Autodesk Inventor part; units mm, degrees
(part 2 of 2)
  line L89 (15.0406, 0.6529) -> (15.0498, 0.6529)
  line L90 (15.0498, 0.6529) -> (15.0498, 0.478)
  spline S139 degree 2 poles (15.0498, 0.478) (15.022, 0.4666) (14.9377, 0.4337) (14.9047, 0.4244) knots 0 0 0 1 2 2 2
  spline S140 degree 2 poles (14.9047, 0.4244) (14.8584, 0.4111) (14.7822, 0.3977) (14.7246, 0.3977) knots 0 0 0 1 2 2 2
  spline S141 degree 2 poles (14.9109, 1.0018) (14.9088, 1.0666) (14.8821, 1.1613) (14.8563, 1.1932) knots 0 0 0 1 2 2 2
  spline S142 degree 2 poles (14.8563, 1.1932) (14.8286, 1.2293) (14.7411, 1.2673) (14.6762, 1.2673) knots 0 0 0 1 2 2 2
  spline S143 degree 2 poles (14.6762, 1.2673) (14.6124, 1.2673) (14.5229, 1.2293) (14.4858, 1.1922) knots 0 0 0 1 2 2 2
  spline S144 degree 2 poles (14.4858, 1.1922) (14.4498, 1.1541) (14.4128, 1.0625) (14.4076, 1.0018) knots 0 0 0 1 2 2 2
  line L91 (14.4076, 1.0018) -> (14.9109, 1.0018)
  line L92 (16.7099, 0.4193) -> (16.5411, 0.4193)
  line L93 (16.5411, 0.4193) -> (16.5411, 1.0409)
  line L94 (16.5411, 1.0409) -> (15.9565, 1.0409)
  line L95 (15.9565, 1.0409) -> (15.9565, 0.4193)
  line L96 (15.9565, 0.4193) -> (15.7878, 0.4193)
  line L97 (15.7878, 0.4193) -> (15.7878, 1.6893)
  line L98 (15.7878, 1.6893) -> (15.9565, 1.6893)
  line L99 (15.9565, 1.6893) -> (15.9565, 1.1912)
  line L100 (15.9565, 1.1912) -> (16.5411, 1.1912)
  line L101 (16.5411, 1.1912) -> (16.5411, 1.6893)
  line L102 (16.5411, 1.6893) -> (16.7099, 1.6893)
  line L103 (16.7099, 1.6893) -> (16.7099, 0.4193)
  line L104 (17.1185, 0.4193) -> (16.9579, 0.4193)
  line L105 (16.9579, 0.4193) -> (16.9579, 1.3723)
  line L106 (16.9579, 1.3723) -> (17.1185, 1.3723)
  line L107 (17.1185, 1.3723) -> (17.1185, 0.4193)
  line L108 (17.1298, 1.5308) -> (16.9476, 1.5308)
  line L109 (16.9476, 1.5308) -> (16.9476, 1.6975)
  line L110 (16.9476, 1.6975) -> (17.1298, 1.6975)
  line L111 (17.1298, 1.6975) -> (17.1298, 1.5308)
  spline S145 degree 2 poles (17.3881, 0.267) (17.4046, 0.2598) (17.4674, 0.2371) (17.5075, 0.2279) knots 0 0 0 1 2 2 2
  spline S146 degree 2 poles (17.5075, 0.2279) (17.5518, 0.2166) (17.6269, 0.2032) (17.6711, 0.2032) knots 0 0 0 1 2 2 2
  spline S147 degree 2 poles (17.6711, 0.2032) (17.7452, 0.2032) (17.8482, 0.2423) (17.877, 0.2773) knots 0 0 0 1 2 2 2
  spline S148 degree 2 poles (17.877, 0.2773) (17.9048, 0.3123) (17.9264, 0.4039) (17.9264, 0.4625) knots 0 0 0 1 2 2 2
  line L112 (17.9264, 0.4625) -> (17.9264, 0.5459)
  spline S149 degree 2 poles (17.9264, 0.5459) (17.8615, 0.4893) (17.737, 0.4358) (17.6434, 0.4358) knots 0 0 0 1 2 2 2
  spline S150 degree 2 poles (17.6434, 0.4358) (17.4807, 0.4358) (17.2883, 0.6776) (17.2883, 0.9051) knots 0 0 0 1 2 2 2
  spline S151 degree 2 poles (17.2883, 0.9051) (17.2883, 1.0234) (17.3552, 1.2066) (17.4108, 1.2715) knots 0 0 0 1 2 2 2
  spline S152 degree 2 poles (17.4108, 1.2715) (17.4643, 1.3322) (17.6114, 1.3991) (17.6897, 1.3991) knots 0 0 0 1 2 2 2
  spline S153 degree 2 poles (17.6897, 1.3991) (17.7638, 1.3991) (17.8718, 1.3641) (17.9264, 1.3322) knots 0 0 0 1 2 2 2
  line L113 (17.9264, 1.3322) -> (17.9356, 1.3723)
  line L114 (17.9356, 1.3723) -> (18.0869, 1.3723)
  line L115 (18.0869, 1.3723) -> (18.0869, 0.5284)
  spline S154 degree 2 poles (18.0869, 0.5284) (18.0869, 0.2855) (17.8759, 0.0591) (17.6588, 0.0591) knots 0 0 0 1 2 2 2
  spline S155 degree 2 poles (17.6588, 0.0591) (17.5888, 0.0591) (17.4427, 0.0817) (17.3799, 0.1003) knots 0 0 0 1 2 2 2
  line L116 (17.3799, 0.1003) -> (17.3799, 0.267)
  line L117 (17.3799, 0.267) -> (17.3881, 0.267)
  line L118 (17.9264, 0.6776) -> (17.9264, 1.2015)
  spline S156 degree 2 poles (17.9264, 1.2015) (17.8667, 1.2303) (17.7658, 1.255) (17.7154, 1.255) knots 0 0 0 1 2 2 2
  spline S157 degree 2 poles (17.7154, 1.255) (17.5939, 1.255) (17.454, 1.0759) (17.454, 0.9082) knots 0 0 0 1 2 2 2
  spline S158 degree 2 poles (17.454, 0.9082) (17.454, 0.7497) (17.56, 0.584) (17.6794, 0.584) knots 0 0 0 1 2 2 2
  spline S159 degree 2 poles (17.6794, 0.584) (17.7422, 0.584) (17.8739, 0.6334) (17.9264, 0.6776) knots 0 0 0 1 2 2 2
  line L119 (19.0677, 0.4193) -> (18.9072, 0.4193)
  line L120 (18.9072, 0.4193) -> (18.9072, 0.9627)
  spline S160 degree 2 poles (18.9072, 0.9627) (18.9072, 1.0286) (18.8948, 1.1418) (18.8763, 1.1757) knots 0 0 0 1 2 2 2
  spline S161 degree 2 poles (18.8763, 1.1757) (18.8567, 1.2118) (18.7868, 1.2468) (18.7271, 1.2468) knots 0 0 0 1 2 2 2
  spline S162 degree 2 poles (18.7271, 1.2468) (18.6674, 1.2468) (18.5408, 1.1829) (18.4801, 1.1315) knots 0 0 0 1 2 2 2
  line L121 (18.4801, 1.1315) -> (18.4801, 0.4193)
  line L122 (18.4801, 0.4193) -> (18.3195, 0.4193)
  line L123 (18.3195, 0.4193) -> (18.3195, 1.7459)
  line L124 (18.3195, 1.7459) -> (18.4801, 1.7459)
  line L125 (18.4801, 1.7459) -> (18.4801, 1.2663)
  spline S163 degree 2 poles (18.4801, 1.2663) (18.5521, 1.3311) (18.691, 1.3991) (18.7693, 1.3991) knots 0 0 0 1 2 2 2
  spline S164 degree 2 poles (18.7693, 1.3991) (18.9092, 1.3991) (19.0677, 1.2138) (19.0677, 1.0378) knots 0 0 0 1 2 2 2
  line L126 (19.0677, 1.0378) -> (19.0677, 0.4193)
  spline S165 degree 2 poles (20.205, 0.3967) (20.0671, 0.3967) (19.8736, 0.4543) (19.7881, 0.4955) knots 0 0 0 1 2 2 2
  line L127 (19.7881, 0.4955) -> (19.7881, 0.7075)
  line L128 (19.7881, 0.7075) -> (19.8005, 0.7075)
  spline S166 degree 2 poles (19.8005, 0.7075) (19.8839, 0.6292) (20.0948, 0.5428) (20.1926, 0.5428) knots 0 0 0 1 2 2 2
  spline S167 degree 2 poles (20.1926, 0.5428) (20.3326, 0.5428) (20.4756, 0.6591) (20.4756, 0.7548) knots 0 0 0 1 2 2 2
  spline S168 degree 2 poles (20.4756, 0.7548) (20.4756, 0.831) (20.4005, 0.9257) (20.3192, 0.9493) knots 0 0 0 1 2 2 2
  spline S169 degree 2 poles (20.3192, 0.9493) (20.2605, 0.9658) (20.1628, 0.9884) (20.0897, 1.007) knots 0 0 0 1 2 2 2
  spline S170 degree 2 poles (20.0897, 1.007) (20.0238, 1.0245) (19.9199, 1.0769) (19.8797, 1.1191) knots 0 0 0 1 2 2 2
  spline S171 degree 2 poles (19.8797, 1.1191) (19.8406, 1.1613) (19.7974, 1.2745) (19.7974, 1.3486) knots 0 0 0 1 2 2 2
  spline S172 degree 2 poles (19.7974, 1.3486) (19.7974, 1.503) (20.0382, 1.7119) (20.2245, 1.7119) knots 0 0 0 1 2 2 2
  spline S173 degree 2 poles (20.2245, 1.7119) (20.3316, 1.7119) (20.5209, 1.6697) (20.6022, 1.6296) knots 0 0 0 1 2 2 2
  line L129 (20.6022, 1.6296) -> (20.6022, 1.4279)
  line L130 (20.6022, 1.4279) -> (20.5899, 1.4279)
  spline S174 degree 2 poles (20.5899, 1.4279) (20.5292, 1.4835) (20.3398, 1.5658) (20.2358, 1.5658) knots 0 0 0 1 2 2 2
  spline S175 degree 2 poles (20.2358, 1.5658) (20.1185, 1.5658) (19.9734, 1.4557) (19.9734, 1.3661) knots 0 0 0 1 2 2 2
  spline S176 degree 2 poles (19.9734, 1.3661) (19.9734, 1.2859) (20.0588, 1.1901) (20.1391, 1.1685) knots 0 0 0 1 2 2 2
  spline S177 degree 2 poles (20.1391, 1.1685) (20.1926, 1.1541) (20.348, 1.1171) (20.3995, 1.1016) knots 0 0 0 1 2 2 2
  spline S178 degree 2 poles (20.3995, 1.1016) (20.5302, 1.0615) (20.6516, 0.8999) (20.6516, 0.7816) knots 0 0 0 1 2 2 2
  spline S179 degree 2 poles (20.6516, 0.7816) (20.6516, 0.7064) (20.5909, 0.5624) (20.5364, 0.5119) knots 0 0 0 1 2 2 2
  spline S180 degree 2 poles (20.5364, 0.5119) (20.4756, 0.4563) (20.3213, 0.3967) (20.205, 0.3967) knots 0 0 0 1 2 2 2
  spline S181 degree 2 poles (21.1899, 0.3977) (21.0911, 0.3977) (20.9274, 0.4584) (20.8688, 0.5202) knots 0 0 0 1 2 2 2
  spline S182 degree 2 poles (20.8688, 0.5202) (20.8101, 0.5809) (20.7453, 0.7682) (20.7453, 0.8937) knots 0 0 0 1 2 2 2
  spline S183 degree 2 poles (20.7453, 0.8937) (20.7453, 1.0193) (20.8122, 1.2025) (20.8688, 1.2642) knots 0 0 0 1 2 2 2
  spline S184 degree 2 poles (20.8688, 1.2642) (20.9254, 1.327) (21.0931, 1.3939) (21.1899, 1.3939) knots 0 0 0 1 2 2 2
  spline S185 degree 2 poles (21.1899, 1.3939) (21.2681, 1.3939) (21.4142, 1.3497) (21.4708, 1.3209) knots 0 0 0 1 2 2 2
  line L131 (21.4708, 1.3209) -> (21.4708, 1.1407)
  line L132 (21.4708, 1.1407) -> (21.4616, 1.1407)
  spline S186 degree 2 poles (21.4616, 1.1407) (21.4441, 1.1552) (21.3906, 1.1922) (21.3525, 1.2118) knots 0 0 0 1 2 2 2
  spline S187 degree 2 poles (21.3525, 1.2118) (21.3185, 1.2282) (21.228, 1.254) (21.1868, 1.254) knots 0 0 0 1 2 2 2
  spline S188 degree 2 poles (21.1868, 1.254) (21.0623, 1.254) (20.911, 1.0656) (20.911, 0.8937) knots 0 0 0 1 2 2 2
  spline S189 degree 2 poles (20.911, 0.8937) (20.911, 0.726) (21.0571, 0.5377) (21.1868, 0.5377) knots 0 0 0 1 2 2 2
  spline S190 degree 2 poles (21.1868, 0.5377) (21.265, 0.5377) (21.407, 0.6025) (21.4616, 0.6529) knots 0 0 0 1 2 2 2
  line L133 (21.4616, 0.6529) -> (21.4708, 0.6529)
  line L134 (21.4708, 0.6529) -> (21.4708, 0.4728)
  spline S191 degree 2 poles (21.4708, 0.4728) (21.4472, 0.4615) (21.3751, 0.4296) (21.3463, 0.4224) knots 0 0 0 1 2 2 2
  spline S192 degree 2 poles (21.3463, 0.4224) (21.3051, 0.41) (21.2403, 0.3977) (21.1899, 0.3977) knots 0 0 0 1 2 2 2
  line L135 (22.3652, 0.4193) -> (22.2046, 0.4193)
  line L136 (22.2046, 0.4193) -> (22.2046, 0.9627)
  spline S193 degree 2 poles (22.2046, 0.9627) (22.2046, 1.0286) (22.1923, 1.1418) (22.1738, 1.1757) knots 0 0 0 1 2 2 2
  spline S194 degree 2 poles (22.1738, 1.1757) (22.1542, 1.2118) (22.0842, 1.2468) (22.0245, 1.2468) knots 0 0 0 1 2 2 2
  spline S195 degree 2 poles (22.0245, 1.2468) (21.9648, 1.2468) (21.8383, 1.1829) (21.7775, 1.1315) knots 0 0 0 1 2 2 2
  line L137 (21.7775, 1.1315) -> (21.7775, 0.4193)
  line L138 (21.7775, 0.4193) -> (21.617, 0.4193)
  line L139 (21.617, 0.4193) -> (21.617, 1.7459)
  line L140 (21.617, 1.7459) -> (21.7775, 1.7459)
  line L141 (21.7775, 1.7459) -> (21.7775, 1.2663)
  spline S196 degree 2 poles (21.7775, 1.2663) (21.8496, 1.3311) (21.9885, 1.3991) (22.0667, 1.3991) knots 0 0 0 1 2 2 2
  spline S197 degree 2 poles (22.0667, 1.3991) (22.2067, 1.3991) (22.3652, 1.2138) (22.3652, 1.0378) knots 0 0 0 1 2 2 2
  line L142 (22.3652, 1.0378) -> (22.3652, 0.4193)
  spline S198 degree 2 poles (23.3738, 0.8958) (23.3738, 0.655) (23.1422, 0.3925) (22.9487, 0.3925) knots 0 0 0 1 2 2 2
  spline S199 degree 2 poles (22.9487, 0.3925) (22.7501, 0.3925) (22.5227, 0.6632) (22.5227, 0.8958) knots 0 0 0 1 2 2 2
  spline S200 degree 2 poles (22.5227, 0.8958) (22.5227, 1.1346) (22.7573, 1.3991) (22.9487, 1.3991) knots 0 0 0 1 2 2 2
  spline S201 degree 2 poles (22.9487, 1.3991) (23.1422, 1.3991) (23.3738, 1.1356) (23.3738, 0.8958) knots 0 0 0 1 2 2 2
  spline S202 degree 2 poles (23.2081, 0.8958) (23.2081, 1.0811) (23.0733, 1.2612) (22.9487, 1.2612) knots 0 0 0 1 2 2 2
  spline S203 degree 2 poles (22.9487, 1.2612) (22.8242, 1.2612) (22.6884, 1.0811) (22.6884, 0.8958) knots 0 0 0 1 2 2 2
  spline S204 degree 2 poles (22.6884, 0.8958) (22.6884, 0.7157) (22.8242, 0.5304) (22.9487, 0.5304) knots 0 0 0 1 2 2 2
  spline S205 degree 2 poles (22.9487, 0.5304) (23.0722, 0.5304) (23.2081, 0.7126) (23.2081, 0.8958) knots 0 0 0 1 2 2 2
  spline S206 degree 2 poles (24.3217, 0.8958) (24.3217, 0.655) (24.0901, 0.3925) (23.8966, 0.3925) knots 0 0 0 1 2 2 2
  spline S207 degree 2 poles (23.8966, 0.3925) (23.698, 0.3925) (23.4705, 0.6632) (23.4705, 0.8958) knots 0 0 0 1 2 2 2
  spline S208 degree 2 poles (23.4705, 0.8958) (23.4705, 1.1346) (23.7052, 1.3991) (23.8966, 1.3991) knots 0 0 0 1 2 2 2
  spline S209 degree 2 poles (23.8966, 1.3991) (24.0901, 1.3991) (24.3217, 1.1356) (24.3217, 0.8958) knots 0 0 0 1 2 2 2
  spline S210 degree 2 poles (24.156, 0.8958) (24.156, 1.0811) (24.0211, 1.2612) (23.8966, 1.2612) knots 0 0 0 1 2 2 2
  spline S211 degree 2 poles (23.8966, 1.2612) (23.7721, 1.2612) (23.6362, 1.0811) (23.6362, 0.8958) knots 0 0 0 1 2 2 2
  spline S212 degree 2 poles (23.6362, 0.8958) (23.6362, 0.7157) (23.7721, 0.5304) (23.8966, 0.5304) knots 0 0 0 1 2 2 2
  spline S213 degree 2 poles (23.8966, 0.5304) (24.0201, 0.5304) (24.156, 0.7126) (24.156, 0.8958) knots 0 0 0 1 2 2 2
  line L143 (24.65, 0.4193) -> (24.4894, 0.4193)
  line L144 (24.4894, 0.4193) -> (24.4894, 1.7459)
  line L145 (24.4894, 1.7459) -> (24.65, 1.7459)
  line L146 (24.65, 1.7459) -> (24.65, 0.4193)
  point P0 (0, 5.7603)
  constraints: 2 other
sketch "Sketch8" plane through (0, 6.6514, 76.2) normal (0.8660254, 0.5, 0) x (0, 0, -1)
  line L0 (0.292, -9.6551) -> (39.862, -9.6551) construction
  line L1 (39.862, -9.6551) -> (39.862, -11.2322) construction
  line L2 (39.862, -11.2322) -> (0.292, -11.2322) construction
  line L3 (0.292, -11.2322) -> (0.292, -9.6551) construction
  spline S0 degree 2 poles (1.775, -10.4157) (1.775, -10.534) (1.7102, -10.7553) (1.6495, -10.8469) knots 0 0 0 1 2 2 2
  line L4 (1.6495, -10.8469) -> (1.2913, -10.8469)
  line L5 (1.2913, -10.8469) -> (1.2697, -10.7481)
  spline S1 degree 2 poles (1.2697, -10.7481) (1.2121, -10.7964) (1.1163, -10.8541) (1.033, -10.8541) knots 0 0 0 1 2 2 2
  spline S2 degree 2 poles (1.033, -10.8541) (0.9023, -10.8541) (0.7345, -10.6431) (0.7345, -10.4434) knots 0 0 0 1 2 2 2
  spline S3 degree 2 poles (0.7345, -10.4434) (0.7345, -10.2428) (0.9404, -10.0194) (1.0731, -10.0194) knots 0 0 0 1 2 2 2
  spline S4 degree 2 poles (1.0731, -10.0194) (1.1349, -10.0194) (1.2234, -10.0503) (1.2687, -10.076) knots 0 0 0 1 2 2 2
  line L6 (1.2687, -10.076) -> (1.2687, -10.0349)
  line L7 (1.2687, -10.0349) -> (1.4035, -10.0349)
  line L8 (1.4035, -10.0349) -> (1.4035, -10.7522)
  line L9 (1.4035, -10.7522) -> (1.597, -10.7522)
  spline S5 degree 2 poles (1.597, -10.7522) (1.6299, -10.6915) (1.6577, -10.499) (1.6577, -10.4208) knots 0 0 0 1 2 2 2
  spline S6 degree 2 poles (1.6577, -10.4208) (1.6577, -10.1419) (1.3736, -9.8023) (1.1071, -9.8023) knots 0 0 0 1 2 2 2
  spline S7 degree 2 poles (1.1071, -9.8023) (0.8549, -9.8023) (0.5266, -10.1697) (0.5266, -10.4321) knots 0 0 0 1 2 2 2
  spline S8 degree 2 poles (0.5266, -10.4321) (0.5266, -10.7131) (0.8457, -11.062) (1.103, -11.062) knots 0 0 0 1 2 2 2
  spline S9 degree 2 poles (1.103, -11.062) (1.1719, -11.062) (1.3253, -11.0434) (1.3932, -11.0229) knots 0 0 0 1 2 2 2
  line L10 (1.3932, -11.0229) -> (1.3932, -11.1433)
  spline S10 degree 2 poles (1.3932, -11.1433) (1.3211, -11.1608) (1.174, -11.1742) (1.1019, -11.1742) knots 0 0 0 1 2 2 2
  spline S11 degree 2 poles (1.1019, -11.1742) (0.8004, -11.1742) (0.4042, -10.7594) (0.4042, -10.4301) knots 0 0 0 1 2 2 2
  spline S12 degree 2 poles (0.4042, -10.4301) (0.4042, -10.1172) (0.8127, -9.687) (1.106, -9.687) knots 0 0 0 1 2 2 2
  spline S13 degree 2 poles (1.106, -9.687) (1.4199, -9.687) (1.775, -10.0915) (1.775, -10.4157) knots 0 0 0 1 2 2 2
  line L11 (1.2666, -10.6338) -> (1.2666, -10.1923)
  spline S14 degree 2 poles (1.2666, -10.1923) (1.2193, -10.1676) (1.139, -10.146) (1.0947, -10.146) knots 0 0 0 1 2 2 2
  spline S15 degree 2 poles (1.0947, -10.146) (0.998, -10.146) (0.8807, -10.2901) (0.8807, -10.4414) knots 0 0 0 1 2 2 2
  spline S16 degree 2 poles (0.8807, -10.4414) (0.8807, -10.5772) (0.9692, -10.7223) (1.0669, -10.7223) knots 0 0 0 1 2 2 2
  spline S17 degree 2 poles (1.0669, -10.7223) (1.1184, -10.7223) (1.2203, -10.6729) (1.2666, -10.6338) knots 0 0 0 1 2 2 2
  line L12 (3.0975, -10.9817) -> (2.9287, -10.9817)
  line L13 (2.9287, -10.9817) -> (2.9287, -9.8877)
  line L14 (2.9287, -9.8877) -> (2.5973, -10.6318)
  line L15 (2.5973, -10.6318) -> (2.4944, -10.6318)
  line L16 (2.4944, -10.6318) -> (2.1661, -9.8877)
  line L17 (2.1661, -9.8877) -> (2.1661, -10.9817)
  line L18 (2.1661, -10.9817) -> (2.0086, -10.9817)
  line L19 (2.0086, -10.9817) -> (2.0086, -9.7117)
  line L20 (2.0086, -9.7117) -> (2.2392, -9.7117)
  line L21 (2.2392, -9.7117) -> (2.5562, -10.4187)
  line L22 (2.5562, -10.4187) -> (2.8628, -9.7117)
  line L23 (2.8628, -9.7117) -> (3.0975, -9.7117)
  line L24 (3.0975, -9.7117) -> (3.0975, -10.9817)
  line L25 (3.5061, -10.9817) -> (3.3455, -10.9817)
  line L26 (3.3455, -10.9817) -> (3.3455, -10.0287)
  line L27 (3.3455, -10.0287) -> (3.5061, -10.0287)
  line L28 (3.5061, -10.0287) -> (3.5061, -10.9817)
  line L29 (3.5174, -9.8702) -> (3.3352, -9.8702)
  line L30 (3.3352, -9.8702) -> (3.3352, -9.7035)
  line L31 (3.3352, -9.7035) -> (3.5174, -9.7035)
  line L32 (3.5174, -9.7035) -> (3.5174, -9.8702)
  spline S18 degree 2 poles (3.9991, -11.0043) (3.9033, -11.0043) (3.7376, -10.9529) (3.6831, -10.9241) knots 0 0 0 1 2 2 2
  line L33 (3.6831, -10.9241) -> (3.6831, -10.744)
  line L34 (3.6831, -10.744) -> (3.6913, -10.744)
  spline S19 degree 2 poles (3.6913, -10.744) (3.7119, -10.7604) (3.7675, -10.7995) (3.8138, -10.8211) knots 0 0 0 1 2 2 2
  spline S20 degree 2 poles (3.8138, -10.8211) (3.8539, -10.8407) (3.9527, -10.8695) (4.0052, -10.8695) knots 0 0 0 1 2 2 2
  spline S21 degree 2 poles (4.0052, -10.8695) (4.0433, -10.8695) (4.1308, -10.852) (4.1514, -10.8376) knots 0 0 0 1 2 2 2
  spline S22 degree 2 poles (4.1514, -10.8376) (4.1812, -10.8181) (4.208, -10.7738) (4.208, -10.7285) knots 0 0 0 1 2 2 2
  spline S23 degree 2 poles (4.208, -10.7285) (4.208, -10.6719) (4.1462, -10.6133) (4.067, -10.5937) knots 0 0 0 1 2 2 2
  spline S24 degree 2 poles (4.067, -10.5937) (4.0361, -10.5865) (3.9373, -10.5659) (3.8951, -10.5546) knots 0 0 0 1 2 2 2
  spline S25 degree 2 poles (3.8951, -10.5546) (3.786, -10.5227) (3.6872, -10.391) (3.6872, -10.2973) knots 0 0 0 1 2 2 2
  spline S26 degree 2 poles (3.6872, -10.2973) (3.6872, -10.1676) (3.8817, -10.006) (4.0423, -10.006) knots 0 0 0 1 2 2 2
  spline S27 degree 2 poles (4.0423, -10.006) (4.1215, -10.006) (4.2821, -10.0451) (4.3366, -10.075) knots 0 0 0 1 2 2 2
  line L35 (4.3366, -10.075) -> (4.3366, -10.2469)
  line L36 (4.3366, -10.2469) -> (4.3284, -10.2469)
  spline S28 degree 2 poles (4.3284, -10.2469) (4.2666, -10.1975) (4.1164, -10.1409) (4.0392, -10.1409) knots 0 0 0 1 2 2 2
  spline S29 degree 2 poles (4.0392, -10.1409) (3.9599, -10.1409) (3.8509, -10.2078) (3.8509, -10.2747) knots 0 0 0 1 2 2 2
  spline S30 degree 2 poles (3.8509, -10.2747) (3.8509, -10.3354) (3.9157, -10.394) (3.9877, -10.4126) knots 0 0 0 1 2 2 2
  spline S31 degree 2 poles (3.9877, -10.4126) (4.0227, -10.4218) (4.1112, -10.4404) (4.1596, -10.4517) knots 0 0 0 1 2 2 2
  spline S32 degree 2 poles (4.1596, -10.4517) (4.2646, -10.4784) (4.3716, -10.6009) (4.3716, -10.7069) knots 0 0 0 1 2 2 2
  spline S33 degree 2 poles (4.3716, -10.7069) (4.3716, -10.7687) (4.3232, -10.8778) (4.2759, -10.9179) knots 0 0 0 1 2 2 2
  spline S34 degree 2 poles (4.2759, -10.9179) (4.2255, -10.9601) (4.0968, -11.0043) (3.9991, -11.0043) knots 0 0 0 1 2 2 2
  spline S35 degree 2 poles (4.7781, -11.0043) (4.6824, -11.0043) (4.5167, -10.9529) (4.4622, -10.9241) knots 0 0 0 1 2 2 2
  line L37 (4.4622, -10.9241) -> (4.4622, -10.744)
  line L38 (4.4622, -10.744) -> (4.4704, -10.744)
  spline S36 degree 2 poles (4.4704, -10.744) (4.491, -10.7604) (4.5466, -10.7995) (4.5929, -10.8211) knots 0 0 0 1 2 2 2
  spline S37 degree 2 poles (4.5929, -10.8211) (4.633, -10.8407) (4.7318, -10.8695) (4.7843, -10.8695) knots 0 0 0 1 2 2 2
  spline S38 degree 2 poles (4.7843, -10.8695) (4.8224, -10.8695) (4.9099, -10.852) (4.9305, -10.8376) knots 0 0 0 1 2 2 2
  spline S39 degree 2 poles (4.9305, -10.8376) (4.9603, -10.8181) (4.9871, -10.7738) (4.9871, -10.7285) knots 0 0 0 1 2 2 2
  spline S40 degree 2 poles (4.9871, -10.7285) (4.9871, -10.6719) (4.9253, -10.6133) (4.8461, -10.5937) knots 0 0 0 1 2 2 2
  spline S41 degree 2 poles (4.8461, -10.5937) (4.8152, -10.5865) (4.7164, -10.5659) (4.6742, -10.5546) knots 0 0 0 1 2 2 2
  spline S42 degree 2 poles (4.6742, -10.5546) (4.5651, -10.5227) (4.4663, -10.391) (4.4663, -10.2973) knots 0 0 0 1 2 2 2
  spline S43 degree 2 poles (4.4663, -10.2973) (4.4663, -10.1676) (4.6608, -10.006) (4.8214, -10.006) knots 0 0 0 1 2 2 2
  spline S44 degree 2 poles (4.8214, -10.006) (4.9006, -10.006) (5.0612, -10.0451) (5.1157, -10.075) knots 0 0 0 1 2 2 2
  line L39 (5.1157, -10.075) -> (5.1157, -10.2469)
  line L40 (5.1157, -10.2469) -> (5.1075, -10.2469)
  spline S45 degree 2 poles (5.1075, -10.2469) (5.0457, -10.1975) (4.8955, -10.1409) (4.8183, -10.1409) knots 0 0 0 1 2 2 2
  spline S46 degree 2 poles (4.8183, -10.1409) (4.739, -10.1409) (4.6299, -10.2078) (4.6299, -10.2747) knots 0 0 0 1 2 2 2
  spline S47 degree 2 poles (4.6299, -10.2747) (4.6299, -10.3354) (4.6948, -10.394) (4.7668, -10.4126) knots 0 0 0 1 2 2 2
  spline S48 degree 2 poles (4.7668, -10.4126) (4.8018, -10.4218) (4.8903, -10.4404) (4.9387, -10.4517) knots 0 0 0 1 2 2 2
  spline S49 degree 2 poles (4.9387, -10.4517) (5.0437, -10.4784) (5.1507, -10.6009) (5.1507, -10.7069) knots 0 0 0 1 2 2 2
  spline S50 degree 2 poles (5.1507, -10.7069) (5.1507, -10.7687) (5.1023, -10.8778) (5.055, -10.9179) knots 0 0 0 1 2 2 2
  spline S51 degree 2 poles (5.055, -10.9179) (5.0046, -10.9601) (4.8759, -11.0043) (4.7781, -11.0043) knots 0 0 0 1 2 2 2
  line L41 (5.4636, -10.9817) -> (5.303, -10.9817)
  line L42 (5.303, -10.9817) -> (5.303, -10.0287)
  line L43 (5.303, -10.0287) -> (5.4636, -10.0287)
  line L44 (5.4636, -10.0287) -> (5.4636, -10.9817)
  line L45 (5.4749, -9.8702) -> (5.2927, -9.8702)
  line L46 (5.2927, -9.8702) -> (5.2927, -9.7035)
  line L47 (5.2927, -9.7035) -> (5.4749, -9.7035)
  line L48 (5.4749, -9.7035) -> (5.4749, -9.8702)
  spline S52 degree 2 poles (6.4825, -10.5052) (6.4825, -10.746) (6.2509, -11.0085) (6.0574, -11.0085) knots 0 0 0 1 2 2 2
  spline S53 degree 2 poles (6.0574, -11.0085) (5.8588, -11.0085) (5.6313, -10.7378) (5.6313, -10.5052) knots 0 0 0 1 2 2 2
  spline S54 degree 2 poles (5.6313, -10.5052) (5.6313, -10.2664) (5.866, -10.0019) (6.0574, -10.0019) knots 0 0 0 1 2 2 2
  spline S55 degree 2 poles (6.0574, -10.0019) (6.2509, -10.0019) (6.4825, -10.2654) (6.4825, -10.5052) knots 0 0 0 1 2 2 2
  spline S56 degree 2 poles (6.3168, -10.5052) (6.3168, -10.3199) (6.1819, -10.1398) (6.0574, -10.1398) knots 0 0 0 1 2 2 2
  spline S57 degree 2 poles (6.0574, -10.1398) (5.9329, -10.1398) (5.797, -10.3199) (5.797, -10.5052) knots 0 0 0 1 2 2 2
  spline S58 degree 2 poles (5.797, -10.5052) (5.797, -10.6853) (5.9329, -10.8705) (6.0574, -10.8705) knots 0 0 0 1 2 2 2
  spline S59 degree 2 poles (6.0574, -10.8705) (6.1809, -10.8705) (6.3168, -10.6884) (6.3168, -10.5052) knots 0 0 0 1 2 2 2
  line L49 (7.3953, -10.9817) -> (7.2348, -10.9817)
  line L50 (7.2348, -10.9817) -> (7.2348, -10.4383)
  spline S60 degree 2 poles (7.2348, -10.4383) (7.2348, -10.3724) (7.2224, -10.2592) (7.2039, -10.2253) knots 0 0 0 1 2 2 2
  spline S61 degree 2 poles (7.2039, -10.2253) (7.1843, -10.1892) (7.1144, -10.1542) (7.0547, -10.1542) knots 0 0 0 1 2 2 2
  spline S62 degree 2 poles (7.0547, -10.1542) (6.995, -10.1542) (6.8684, -10.2181) (6.8077, -10.2695) knots 0 0 0 1 2 2 2
  line L51 (6.8077, -10.2695) -> (6.8077, -10.9817)
  line L52 (6.8077, -10.9817) -> (6.6471, -10.9817)
  line L53 (6.6471, -10.9817) -> (6.6471, -10.0287)
  line L54 (6.6471, -10.0287) -> (6.8077, -10.0287)
  line L55 (6.8077, -10.0287) -> (6.8077, -10.1347)
  spline S63 degree 2 poles (6.8077, -10.1347) (6.8797, -10.0699) (7.0187, -10.0019) (7.0969, -10.0019) knots 0 0 0 1 2 2 2
  spline S64 degree 2 poles (7.0969, -10.0019) (7.2368, -10.0019) (7.3953, -10.1872) (7.3953, -10.3632) knots 0 0 0 1 2 2 2
  line L56 (7.3953, -10.3632) -> (7.3953, -10.9817)
  spline S65 degree 2 poles (8.5326, -11.0043) (8.3947, -11.0043) (8.2012, -10.9467) (8.1157, -10.9055) knots 0 0 0 1 2 2 2
  line L57 (8.1157, -10.9055) -> (8.1157, -10.6935)
  line L58 (8.1157, -10.6935) -> (8.1281, -10.6935)
  spline S66 degree 2 poles (8.1281, -10.6935) (8.2115, -10.7717) (8.4224, -10.8582) (8.5202, -10.8582) knots 0 0 0 1 2 2 2
  spline S67 degree 2 poles (8.5202, -10.8582) (8.6602, -10.8582) (8.8032, -10.7419) (8.8032, -10.6462) knots 0 0 0 1 2 2 2
  spline S68 degree 2 poles (8.8032, -10.6462) (8.8032, -10.57) (8.7281, -10.4753) (8.6468, -10.4517) knots 0 0 0 1 2 2 2
  spline S69 degree 2 poles (8.6468, -10.4517) (8.5881, -10.4352) (8.4904, -10.4126) (8.4173, -10.394) knots 0 0 0 1 2 2 2
  spline S70 degree 2 poles (8.4173, -10.394) (8.3514, -10.3765) (8.2475, -10.3241) (8.2073, -10.2819) knots 0 0 0 1 2 2 2
  spline S71 degree 2 poles (8.2073, -10.2819) (8.1682, -10.2397) (8.125, -10.1265) (8.125, -10.0524) knots 0 0 0 1 2 2 2
  spline S72 degree 2 poles (8.125, -10.0524) (8.125, -9.898) (8.3658, -9.6891) (8.5521, -9.6891) knots 0 0 0 1 2 2 2
  spline S73 degree 2 poles (8.5521, -9.6891) (8.6592, -9.6891) (8.8485, -9.7313) (8.9298, -9.7714) knots 0 0 0 1 2 2 2
  line L59 (8.9298, -9.7714) -> (8.9298, -9.9731)
  line L60 (8.9298, -9.9731) -> (8.9175, -9.9731)
  spline S74 degree 2 poles (8.9175, -9.9731) (8.8568, -9.9175) (8.6674, -9.8352) (8.5634, -9.8352) knots 0 0 0 1 2 2 2
  spline S75 degree 2 poles (8.5634, -9.8352) (8.4461, -9.8352) (8.301, -9.9453) (8.301, -10.0349) knots 0 0 0 1 2 2 2
  spline S76 degree 2 poles (8.301, -10.0349) (8.301, -10.1151) (8.3864, -10.2108) (8.4667, -10.2325) knots 0 0 0 1 2 2 2
  spline S77 degree 2 poles (8.4667, -10.2325) (8.5202, -10.2469) (8.6756, -10.2839) (8.7271, -10.2994) knots 0 0 0 1 2 2 2
  spline S78 degree 2 poles (8.7271, -10.2994) (8.8578, -10.3395) (8.9792, -10.5011) (8.9792, -10.6194) knots 0 0 0 1 2 2 2
  spline S79 degree 2 poles (8.9792, -10.6194) (8.9792, -10.6946) (8.9185, -10.8386) (8.864, -10.8891) knots 0 0 0 1 2 2 2
  spline S80 degree 2 poles (8.864, -10.8891) (8.8032, -10.9446) (8.6489, -11.0043) (8.5326, -11.0043) knots 0 0 0 1 2 2 2
  spline S81 degree 2 poles (9.6698, -10.8808) (9.6502, -10.8952) (9.5844, -10.9467) (9.5535, -10.9621) knots 0 0 0 1 2 2 2
  spline S82 degree 2 poles (9.5535, -10.9621) (9.5113, -10.9848) (9.4321, -11.0085) (9.36, -11.0085) knots 0 0 0 1 2 2 2
  spline S83 degree 2 poles (9.36, -11.0085) (9.3014, -11.0085) (9.1954, -10.9642) (9.1552, -10.9241) knots 0 0 0 1 2 2 2
  spline S84 degree 2 poles (9.1552, -10.9241) (9.1171, -10.885) (9.0708, -10.7697) (9.0708, -10.7059) knots 0 0 0 1 2 2 2
  spline S85 degree 2 poles (9.0708, -10.7059) (9.0708, -10.6071) (9.1542, -10.4671) (9.2448, -10.427) knots 0 0 0 1 2 2 2
  spline S86 degree 2 poles (9.2448, -10.427) (9.325, -10.3899) (9.5432, -10.3621) (9.6698, -10.3549) knots 0 0 0 1 2 2 2
  line L61 (9.6698, -10.3549) -> (9.6698, -10.3241)
  spline S87 degree 2 poles (9.6698, -10.3241) (9.6698, -10.2685) (9.6358, -10.1995) (9.605, -10.18) knots 0 0 0 1 2 2 2
  spline S88 degree 2 poles (9.605, -10.18) (9.5741, -10.1604) (9.4856, -10.1481) (9.4382, -10.1481) knots 0 0 0 1 2 2 2
  spline S89 degree 2 poles (9.4382, -10.1481) (9.3827, -10.1481) (9.2324, -10.181) (9.1573, -10.2129) knots 0 0 0 1 2 2 2
  line L62 (9.1573, -10.2129) -> (9.148, -10.2129)
  line L63 (9.148, -10.2129) -> (9.148, -10.0493)
  spline S90 degree 2 poles (9.148, -10.0493) (9.1923, -10.0369) (9.358, -10.006) (9.4393, -10.006) knots 0 0 0 1 2 2 2
  spline S91 degree 2 poles (9.4393, -10.006) (9.5381, -10.006) (9.6729, -10.0369) (9.7264, -10.0771) knots 0 0 0 1 2 2 2
  spline S92 degree 2 poles (9.7264, -10.0771) (9.7789, -10.1162) (9.8304, -10.2407) (9.8304, -10.3302) knots 0 0 0 1 2 2 2
  line L64 (9.8304, -10.3302) -> (9.8304, -10.9817)
  line L65 (9.8304, -10.9817) -> (9.6698, -10.9817)
  line L66 (9.6698, -10.9817) -> (9.6698, -10.8808)
  line L67 (9.6698, -10.747) -> (9.6698, -10.4825)
  spline S93 degree 2 poles (9.6698, -10.4825) (9.6122, -10.4877) (9.4382, -10.5052) (9.3837, -10.5217) knots 0 0 0 1 2 2 2
  spline S94 degree 2 poles (9.3837, -10.5217) (9.3199, -10.5412) (9.2365, -10.6225) (9.2365, -10.6946) knots 0 0 0 1 2 2 2
  spline S95 degree 2 poles (9.2365, -10.6946) (9.2365, -10.7769) (9.3291, -10.8603) (9.4177, -10.8603) knots 0 0 0 1 2 2 2
  spline S96 degree 2 poles (9.4177, -10.8603) (9.4928, -10.8603) (9.6163, -10.7954) (9.6698, -10.747) knots 0 0 0 1 2 2 2
  line L68 (10.804, -10.9817) -> (10.6434, -10.9817)
  line L69 (10.6434, -10.9817) -> (10.6434, -10.4383)
  spline S97 degree 2 poles (10.6434, -10.4383) (10.6434, -10.3724) (10.631, -10.2592) (10.6125, -10.2253) knots 0 0 0 1 2 2 2
  spline S98 degree 2 poles (10.6125, -10.2253) (10.593, -10.1892) (10.523, -10.1542) (10.4633, -10.1542) knots 0 0 0 1 2 2 2
  spline S99 degree 2 poles (10.4633, -10.1542) (10.4036, -10.1542) (10.277, -10.2181) (10.2163, -10.2695) knots 0 0 0 1 2 2 2
  line L70 (10.2163, -10.2695) -> (10.2163, -10.9817)
  line L71 (10.2163, -10.9817) -> (10.0557, -10.9817)
  line L72 (10.0557, -10.9817) -> (10.0557, -10.0287)
  line L73 (10.0557, -10.0287) -> (10.2163, -10.0287)
  line L74 (10.2163, -10.0287) -> (10.2163, -10.1347)
  spline S100 degree 2 poles (10.2163, -10.1347) (10.2883, -10.0699) (10.4273, -10.0019) (10.5055, -10.0019) knots 0 0 0 1 2 2 2
  spline S101 degree 2 poles (10.5055, -10.0019) (10.6455, -10.0019) (10.804, -10.1872) (10.804, -10.3632) knots 0 0 0 1 2 2 2
  line L75 (10.804, -10.3632) -> (10.804, -10.9817)
  spline S102 degree 2 poles (12.0657, -10.6513) (12.0657, -10.8181) (11.8619, -10.9992) (11.6901, -10.9992) knots 0 0 0 1 2 2 2
  spline S103 degree 2 poles (11.6901, -10.9992) (11.6489, -10.9992) (11.512, -10.9848) (11.4657, -10.9745) knots 0 0 0 1 2 2 2
  line L76 (11.4657, -10.9745) -> (11.4657, -10.8119)
  line L77 (11.4657, -10.8119) -> (11.475, -10.8119)
  spline S104 degree 2 poles (11.475, -10.8119) (11.51, -10.8242) (11.6139, -10.8531) (11.6674, -10.8531) knots 0 0 0 1 2 2 2
  spline S105 degree 2 poles (11.6674, -10.8531) (11.7456, -10.8531) (11.8393, -10.817) (11.8609, -10.7841) knots 0 0 0 1 2 2 2
  spline S106 degree 2 poles (11.8609, -10.7841) (11.8846, -10.7501) (11.8969, -10.6513) (11.8969, -10.5865) knots 0 0 0 1 2 2 2
  line L78 (11.8969, -10.5865) -> (11.8969, -9.8465)
  line L79 (11.8969, -9.8465) -> (11.6283, -9.8465)
  line L80 (11.6283, -9.8465) -> (11.6283, -9.7117)
  line L81 (11.6283, -9.7117) -> (12.0657, -9.7117)
  line L82 (12.0657, -9.7117) -> (12.0657, -10.6513)
  spline S107 degree 2 poles (13.0856, -10.5052) (13.0856, -10.746) (12.8541, -11.0085) (12.6606, -11.0085) knots 0 0 0 1 2 2 2
  spline S108 degree 2 poles (12.6606, -11.0085) (12.4619, -11.0085) (12.2345, -10.7378) (12.2345, -10.5052) knots 0 0 0 1 2 2 2
  spline S109 degree 2 poles (12.2345, -10.5052) (12.2345, -10.2664) (12.4692, -10.0019) (12.6606, -10.0019) knots 0 0 0 1 2 2 2
  spline S110 degree 2 poles (12.6606, -10.0019) (12.8541, -10.0019) (13.0856, -10.2654) (13.0856, -10.5052) knots 0 0 0 1 2 2 2
  spline S111 degree 2 poles (12.9199, -10.5052) (12.9199, -10.3199) (12.7851, -10.1398) (12.6606, -10.1398) knots 0 0 0 1 2 2 2
  spline S112 degree 2 poles (12.6606, -10.1398) (12.536, -10.1398) (12.4002, -10.3199) (12.4002, -10.5052) knots 0 0 0 1 2 2 2
  spline S113 degree 2 poles (12.4002, -10.5052) (12.4002, -10.6853) (12.536, -10.8705) (12.6606, -10.8705) knots 0 0 0 1 2 2 2
  spline S114 degree 2 poles (12.6606, -10.8705) (12.7841, -10.8705) (12.9199, -10.6884) (12.9199, -10.5052) knots 0 0 0 1 2 2 2
  spline S115 degree 2 poles (13.5076, -11.0043) (13.4119, -11.0043) (13.2462, -10.9529) (13.1916, -10.9241) knots 0 0 0 1 2 2 2
  line L83 (13.1916, -10.9241) -> (13.1916, -10.744)
  line L84 (13.1916, -10.744) -> (13.1999, -10.744)
  spline S116 degree 2 poles (13.1999, -10.744) (13.2205, -10.7604) (13.276, -10.7995) (13.3223, -10.8211) knots 0 0 0 1 2 2 2
  spline S117 degree 2 poles (13.3223, -10.8211) (13.3625, -10.8407) (13.4613, -10.8695) (13.5138, -10.8695) knots 0 0 0 1 2 2 2
  spline S118 degree 2 poles (13.5138, -10.8695) (13.5518, -10.8695) (13.6393, -10.852) (13.6599, -10.8376) knots 0 0 0 1 2 2 2
  spline S119 degree 2 poles (13.6599, -10.8376) (13.6898, -10.8181) (13.7165, -10.7738) (13.7165, -10.7285) knots 0 0 0 1 2 2 2
  spline S120 degree 2 poles (13.7165, -10.7285) (13.7165, -10.6719) (13.6548, -10.6133) (13.5755, -10.5937) knots 0 0 0 1 2 2 2
  spline S121 degree 2 poles (13.5755, -10.5937) (13.5446, -10.5865) (13.4458, -10.5659) (13.4036, -10.5546) knots 0 0 0 1 2 2 2
  spline S122 degree 2 poles (13.4036, -10.5546) (13.2946, -10.5227) (13.1957, -10.391) (13.1957, -10.2973) knots 0 0 0 1 2 2 2
  spline S123 degree 2 poles (13.1957, -10.2973) (13.1957, -10.1676) (13.3903, -10.006) (13.5508, -10.006) knots 0 0 0 1 2 2 2
  spline S124 degree 2 poles (13.5508, -10.006) (13.6301, -10.006) (13.7906, -10.0451) (13.8452, -10.075) knots 0 0 0 1 2 2 2
  line L85 (13.8452, -10.075) -> (13.8452, -10.2469)
  line L86 (13.8452, -10.2469) -> (13.8369, -10.2469)
  spline S125 degree 2 poles (13.8369, -10.2469) (13.7752, -10.1975) (13.6249, -10.1409) (13.5477, -10.1409) knots 0 0 0 1 2 2 2
  spline S126 degree 2 poles (13.5477, -10.1409) (13.4685, -10.1409) (13.3594, -10.2078) (13.3594, -10.2747) knots 0 0 0 1 2 2 2
  spline S127 degree 2 poles (13.3594, -10.2747) (13.3594, -10.3354) (13.4242, -10.394) (13.4963, -10.4126) knots 0 0 0 1 2 2 2
  spline S128 degree 2 poles (13.4963, -10.4126) (13.5313, -10.4218) (13.6198, -10.4404) (13.6681, -10.4517) knots 0 0 0 1 2 2 2
  spline S129 degree 2 poles (13.6681, -10.4517) (13.7731, -10.4784) (13.8802, -10.6009) (13.8802, -10.7069) knots 0 0 0 1 2 2 2
  spline S130 degree 2 poles (13.8802, -10.7069) (13.8802, -10.7687) (13.8318, -10.8778) (13.7844, -10.9179) knots 0 0 0 1 2 2 2
  spline S131 degree 2 poles (13.7844, -10.9179) (13.734, -10.9601) (13.6054, -11.0043) (13.5076, -11.0043) knots 0 0 0 1 2 2 2
  spline S132 degree 2 poles (14.4431, -11.0033) (14.2146, -11.0033) (13.9635, -10.747) (13.9635, -10.5103) knots 0 0 0 1 2 2 2
  spline S133 degree 2 poles (13.9635, -10.5103) (13.9635, -10.2777) (14.2074, -10.0019) (14.404, -10.0019) knots 0 0 0 1 2 2 2
  spline S134 degree 2 poles (14.404, -10.0019) (14.4925, -10.0019) (14.6294, -10.0534) (14.6798, -10.1079) knots 0 0 0 1 2 2 2
  spline S135 degree 2 poles (14.6798, -10.1079) (14.7313, -10.1625) (14.7858, -10.3199) (14.7858, -10.4342) knots 0 0 0 1 2 2 2
  line L87 (14.7858, -10.4342) -> (14.7858, -10.5217)
  line L88 (14.7858, -10.5217) -> (14.1261, -10.5217)
  spline S136 degree 2 poles (14.1261, -10.5217) (14.1261, -10.6874) (14.2928, -10.8633) (14.441, -10.8633) knots 0 0 0 1 2 2 2
  spline S137 degree 2 poles (14.441, -10.8633) (14.4935, -10.8633) (14.5954, -10.8397) (14.6366, -10.8211) knots 0 0 0 1 2 2 2
  spline S138 degree 2 poles (14.6366, -10.8211) (14.6798, -10.8006) (14.7395, -10.7645) (14.7591, -10.7481) knots 0 0 0 1 2 2 2
  line L89 (14.7591, -10.7481) -> (14.7683, -10.7481)
  line L90 (14.7683, -10.7481) -> (14.7683, -10.923)
  spline S139 degree 2 poles (14.7683, -10.923) (14.7405, -10.9344) (14.6561, -10.9673) (14.6232, -10.9766) knots 0 0 0 1 2 2 2
  spline S140 degree 2 poles (14.6232, -10.9766) (14.5769, -10.9899) (14.5007, -11.0033) (14.4431, -11.0033) knots 0 0 0 1 2 2 2
  spline S141 degree 2 poles (14.6294, -10.3992) (14.6273, -10.3343) (14.6006, -10.2397) (14.5748, -10.2078) knots 0 0 0 1 2 2 2
  spline S142 degree 2 poles (14.5748, -10.2078) (14.5471, -10.1717) (14.4596, -10.1337) (14.3947, -10.1337) knots 0 0 0 1 2 2 2
  spline S143 degree 2 poles (14.3947, -10.1337) (14.3309, -10.1337) (14.2414, -10.1717) (14.2043, -10.2088) knots 0 0 0 1 2 2 2
  spline S144 degree 2 poles (14.2043, -10.2088) (14.1683, -10.2469) (14.1313, -10.3385) (14.1261, -10.3992) knots 0 0 0 1 2 2 2
  line L91 (14.1261, -10.3992) -> (14.6294, -10.3992)
  line L92 (16.4284, -10.9817) -> (16.2596, -10.9817)
  line L93 (16.2596, -10.9817) -> (16.2596, -10.3601)
  line L94 (16.2596, -10.3601) -> (15.675, -10.3601)
  line L95 (15.675, -10.3601) -> (15.675, -10.9817)
  line L96 (15.675, -10.9817) -> (15.5062, -10.9817)
  line L97 (15.5062, -10.9817) -> (15.5062, -9.7117)
  line L98 (15.5062, -9.7117) -> (15.675, -9.7117)
  line L99 (15.675, -9.7117) -> (15.675, -10.2098)
  line L100 (15.675, -10.2098) -> (16.2596, -10.2098)
  line L101 (16.2596, -10.2098) -> (16.2596, -9.7117)
  line L102 (16.2596, -9.7117) -> (16.4284, -9.7117)
  line L103 (16.4284, -9.7117) -> (16.4284, -10.9817)
  line L104 (16.837, -10.9817) -> (16.6764, -10.9817)
  line L105 (16.6764, -10.9817) -> (16.6764, -10.0287)
  line L106 (16.6764, -10.0287) -> (16.837, -10.0287)
  line L107 (16.837, -10.0287) -> (16.837, -10.9817)
  line L108 (16.8483, -9.8702) -> (16.6661, -9.8702)
  line L109 (16.6661, -9.8702) -> (16.6661, -9.7035)
  line L110 (16.6661, -9.7035) -> (16.8483, -9.7035)
  line L111 (16.8483, -9.7035) -> (16.8483, -9.8702)
  spline S145 degree 2 poles (17.1066, -11.134) (17.1231, -11.1412) (17.1859, -11.1639) (17.226, -11.1731) knots 0 0 0 1 2 2 2
  spline S146 degree 2 poles (17.226, -11.1731) (17.2702, -11.1844) (17.3454, -11.1978) (17.3896, -11.1978) knots 0 0 0 1 2 2 2
  spline S147 degree 2 poles (17.3896, -11.1978) (17.4637, -11.1978) (17.5666, -11.1587) (17.5955, -11.1237) knots 0 0 0 1 2 2 2
  spline S148 degree 2 poles (17.5955, -11.1237) (17.6233, -11.0887) (17.6449, -10.9971) (17.6449, -10.9385) knots 0 0 0 1 2 2 2
  line L112 (17.6449, -10.9385) -> (17.6449, -10.8551)
  spline S149 degree 2 poles (17.6449, -10.8551) (17.58, -10.9117) (17.4555, -10.9652) (17.3618, -10.9652) knots 0 0 0 1 2 2 2
  spline S150 degree 2 poles (17.3618, -10.9652) (17.1992, -10.9652) (17.0068, -10.7234) (17.0068, -10.4959) knots 0 0 0 1 2 2 2
  spline S151 degree 2 poles (17.0068, -10.4959) (17.0068, -10.3776) (17.0737, -10.1944) (17.1293, -10.1295) knots 0 0 0 1 2 2 2
  spline S152 degree 2 poles (17.1293, -10.1295) (17.1828, -10.0688) (17.3299, -10.0019) (17.4082, -10.0019) knots 0 0 0 1 2 2 2
  spline S153 degree 2 poles (17.4082, -10.0019) (17.4823, -10.0019) (17.5903, -10.0369) (17.6449, -10.0688) knots 0 0 0 1 2 2 2
  line L113 (17.6449, -10.0688) -> (17.6541, -10.0287)
  line L114 (17.6541, -10.0287) -> (17.8054, -10.0287)
  line L115 (17.8054, -10.0287) -> (17.8054, -10.8726)
  spline S154 degree 2 poles (17.8054, -10.8726) (17.8054, -11.1155) (17.5944, -11.3419) (17.3773, -11.3419) knots 0 0 0 1 2 2 2
  spline S155 degree 2 poles (17.3773, -11.3419) (17.3073, -11.3419) (17.1612, -11.3193) (17.0984, -11.3007) knots 0 0 0 1 2 2 2
  line L116 (17.0984, -11.3007) -> (17.0984, -11.134)
  line L117 (17.0984, -11.134) -> (17.1066, -11.134)
  line L118 (17.6449, -10.7234) -> (17.6449, -10.1995)
  spline S156 degree 2 poles (17.6449, -10.1995) (17.5852, -10.1707) (17.4843, -10.146) (17.4339, -10.146) knots 0 0 0 1 2 2 2
  spline S157 degree 2 poles (17.4339, -10.146) (17.3124, -10.146) (17.1725, -10.3251) (17.1725, -10.4928) knots 0 0 0 1 2 2 2
  spline S158 degree 2 poles (17.1725, -10.4928) (17.1725, -10.6513) (17.2785, -10.817) (17.3979, -10.817) knots 0 0 0 1 2 2 2
  spline S159 degree 2 poles (17.3979, -10.817) (17.4606, -10.817) (17.5924, -10.7676) (17.6449, -10.7234) knots 0 0 0 1 2 2 2
  line L119 (18.7862, -10.9817) -> (18.6257, -10.9817)
  line L120 (18.6257, -10.9817) -> (18.6257, -10.4383)
  spline S160 degree 2 poles (18.6257, -10.4383) (18.6257, -10.3724) (18.6133, -10.2592) (18.5948, -10.2253) knots 0 0 0 1 2 2 2
  spline S161 degree 2 poles (18.5948, -10.2253) (18.5752, -10.1892) (18.5053, -10.1542) (18.4456, -10.1542) knots 0 0 0 1 2 2 2
  spline S162 degree 2 poles (18.4456, -10.1542) (18.3859, -10.1542) (18.2593, -10.2181) (18.1986, -10.2695) knots 0 0 0 1 2 2 2
  line L121 (18.1986, -10.2695) -> (18.1986, -10.9817)
  line L122 (18.1986, -10.9817) -> (18.038, -10.9817)
  line L123 (18.038, -10.9817) -> (18.038, -9.6551)
  line L124 (18.038, -9.6551) -> (18.1986, -9.6551)
  line L125 (18.1986, -9.6551) -> (18.1986, -10.1347)
  spline S163 degree 2 poles (18.1986, -10.1347) (18.2706, -10.0699) (18.4095, -10.0019) (18.4878, -10.0019) knots 0 0 0 1 2 2 2
  spline S164 degree 2 poles (18.4878, -10.0019) (18.6277, -10.0019) (18.7862, -10.1872) (18.7862, -10.3632) knots 0 0 0 1 2 2 2
  line L126 (18.7862, -10.3632) -> (18.7862, -10.9817)
  spline S165 degree 2 poles (19.9235, -11.0043) (19.7855, -11.0043) (19.5921, -10.9467) (19.5066, -10.9055) knots 0 0 0 1 2 2 2
  line L127 (19.5066, -10.9055) -> (19.5066, -10.6935)
  line L128 (19.5066, -10.6935) -> (19.519, -10.6935)
  spline S166 degree 2 poles (19.519, -10.6935) (19.6024, -10.7717) (19.8133, -10.8582) (19.9111, -10.8582) knots 0 0 0 1 2 2 2
  spline S167 degree 2 poles (19.9111, -10.8582) (20.0511, -10.8582) (20.1941, -10.7419) (20.1941, -10.6462) knots 0 0 0 1 2 2 2
  spline S168 degree 2 poles (20.1941, -10.6462) (20.1941, -10.57) (20.119, -10.4753) (20.0377, -10.4517) knots 0 0 0 1 2 2 2
  spline S169 degree 2 poles (20.0377, -10.4517) (19.979, -10.4352) (19.8813, -10.4126) (19.8082, -10.394) knots 0 0 0 1 2 2 2
  spline S170 degree 2 poles (19.8082, -10.394) (19.7423, -10.3765) (19.6384, -10.3241) (19.5982, -10.2819) knots 0 0 0 1 2 2 2
  spline S171 degree 2 poles (19.5982, -10.2819) (19.5591, -10.2397) (19.5159, -10.1265) (19.5159, -10.0524) knots 0 0 0 1 2 2 2
  spline S172 degree 2 poles (19.5159, -10.0524) (19.5159, -9.898) (19.7567, -9.6891) (19.943, -9.6891) knots 0 0 0 1 2 2 2
  spline S173 degree 2 poles (19.943, -9.6891) (20.05, -9.6891) (20.2394, -9.7313) (20.3207, -9.7714) knots 0 0 0 1 2 2 2
  line L129 (20.3207, -9.7714) -> (20.3207, -9.9731)
  line L130 (20.3207, -9.9731) -> (20.3084, -9.9731)
  spline S174 degree 2 poles (20.3084, -9.9731) (20.2476, -9.9175) (20.0583, -9.8352) (19.9543, -9.8352) knots 0 0 0 1 2 2 2
  spline S175 degree 2 poles (19.9543, -9.8352) (19.837, -9.8352) (19.6919, -9.9453) (19.6919, -10.0349) knots 0 0 0 1 2 2 2
  spline S176 degree 2 poles (19.6919, -10.0349) (19.6919, -10.1151) (19.7773, -10.2108) (19.8576, -10.2325) knots 0 0 0 1 2 2 2
  spline S177 degree 2 poles (19.8576, -10.2325) (19.9111, -10.2469) (20.0665, -10.2839) (20.118, -10.2994) knots 0 0 0 1 2 2 2
  spline S178 degree 2 poles (20.118, -10.2994) (20.2487, -10.3395) (20.3701, -10.5011) (20.3701, -10.6194) knots 0 0 0 1 2 2 2
  spline S179 degree 2 poles (20.3701, -10.6194) (20.3701, -10.6946) (20.3094, -10.8386) (20.2549, -10.8891) knots 0 0 0 1 2 2 2
  spline S180 degree 2 poles (20.2549, -10.8891) (20.1941, -10.9446) (20.0398, -11.0043) (19.9235, -11.0043) knots 0 0 0 1 2 2 2
  spline S181 degree 2 poles (20.9084, -11.0033) (20.8096, -11.0033) (20.6459, -10.9426) (20.5873, -10.8808) knots 0 0 0 1 2 2 2
  spline S182 degree 2 poles (20.5873, -10.8808) (20.5286, -10.8201) (20.4638, -10.6328) (20.4638, -10.5072) knots 0 0 0 1 2 2 2
  spline S183 degree 2 poles (20.4638, -10.5072) (20.4638, -10.3817) (20.5307, -10.1985) (20.5873, -10.1367) knots 0 0 0 1 2 2 2
  spline S184 degree 2 poles (20.5873, -10.1367) (20.6439, -10.074) (20.8116, -10.0071) (20.9084, -10.0071) knots 0 0 0 1 2 2 2
  spline S185 degree 2 poles (20.9084, -10.0071) (20.9866, -10.0071) (21.1327, -10.0513) (21.1893, -10.0801) knots 0 0 0 1 2 2 2
  line L131 (21.1893, -10.0801) -> (21.1893, -10.2602)
  line L132 (21.1893, -10.2602) -> (21.1801, -10.2602)
  spline S186 degree 2 poles (21.1801, -10.2602) (21.1626, -10.2458) (21.1091, -10.2088) (21.071, -10.1892) knots 0 0 0 1 2 2 2
  spline S187 degree 2 poles (21.071, -10.1892) (21.037, -10.1728) (20.9465, -10.147) (20.9053, -10.147) knots 0 0 0 1 2 2 2
  spline S188 degree 2 poles (20.9053, -10.147) (20.7808, -10.147) (20.6295, -10.3354) (20.6295, -10.5072) knots 0 0 0 1 2 2 2
  spline S189 degree 2 poles (20.6295, -10.5072) (20.6295, -10.675) (20.7756, -10.8633) (20.9053, -10.8633) knots 0 0 0 1 2 2 2
  spline S190 degree 2 poles (20.9053, -10.8633) (20.9835, -10.8633) (21.1255, -10.7985) (21.1801, -10.7481) knots 0 0 0 1 2 2 2
  line L133 (21.1801, -10.7481) -> (21.1893, -10.7481)
  line L134 (21.1893, -10.7481) -> (21.1893, -10.9282)
  spline S191 degree 2 poles (21.1893, -10.9282) (21.1657, -10.9395) (21.0936, -10.9714) (21.0648, -10.9786) knots 0 0 0 1 2 2 2
  spline S192 degree 2 poles (21.0648, -10.9786) (21.0236, -10.991) (20.9588, -11.0033) (20.9084, -11.0033) knots 0 0 0 1 2 2 2
  line L135 (22.0837, -10.9817) -> (21.9231, -10.9817)
  line L136 (21.9231, -10.9817) -> (21.9231, -10.4383)
  spline S193 degree 2 poles (21.9231, -10.4383) (21.9231, -10.3724) (21.9108, -10.2592) (21.8923, -10.2253) knots 0 0 0 1 2 2 2
  spline S194 degree 2 poles (21.8923, -10.2253) (21.8727, -10.1892) (21.8027, -10.1542) (21.743, -10.1542) knots 0 0 0 1 2 2 2
  spline S195 degree 2 poles (21.743, -10.1542) (21.6833, -10.1542) (21.5568, -10.2181) (21.496, -10.2695) knots 0 0 0 1 2 2 2
  line L137 (21.496, -10.2695) -> (21.496, -10.9817)
  line L138 (21.496, -10.9817) -> (21.3355, -10.9817)
  line L139 (21.3355, -10.9817) -> (21.3355, -9.6551)
  line L140 (21.3355, -9.6551) -> (21.496, -9.6551)
  line L141 (21.496, -9.6551) -> (21.496, -10.1347)
  spline S196 degree 2 poles (21.496, -10.1347) (21.5681, -10.0699) (21.707, -10.0019) (21.7852, -10.0019) knots 0 0 0 1 2 2 2
  spline S197 degree 2 poles (21.7852, -10.0019) (21.9252, -10.0019) (22.0837, -10.1872) (22.0837, -10.3632) knots 0 0 0 1 2 2 2
  line L142 (22.0837, -10.3632) -> (22.0837, -10.9817)
  spline S198 degree 2 poles (23.0923, -10.5052) (23.0923, -10.746) (22.8607, -11.0085) (22.6672, -11.0085) knots 0 0 0 1 2 2 2
  spline S199 degree 2 poles (22.6672, -11.0085) (22.4686, -11.0085) (22.2412, -10.7378) (22.2412, -10.5052) knots 0 0 0 1 2 2 2
  spline S200 degree 2 poles (22.2412, -10.5052) (22.2412, -10.2664) (22.4758, -10.0019) (22.6672, -10.0019) knots 0 0 0 1 2 2 2
  spline S201 degree 2 poles (22.6672, -10.0019) (22.8607, -10.0019) (23.0923, -10.2654) (23.0923, -10.5052) knots 0 0 0 1 2 2 2
  spline S202 degree 2 poles (22.9266, -10.5052) (22.9266, -10.3199) (22.7918, -10.1398) (22.6672, -10.1398) knots 0 0 0 1 2 2 2
  spline S203 degree 2 poles (22.6672, -10.1398) (22.5427, -10.1398) (22.4069, -10.3199) (22.4069, -10.5052) knots 0 0 0 1 2 2 2
  spline S204 degree 2 poles (22.4069, -10.5052) (22.4069, -10.6853) (22.5427, -10.8705) (22.6672, -10.8705) knots 0 0 0 1 2 2 2
  spline S205 degree 2 poles (22.6672, -10.8705) (22.7907, -10.8705) (22.9266, -10.6884) (22.9266, -10.5052) knots 0 0 0 1 2 2 2
  spline S206 degree 2 poles (24.0402, -10.5052) (24.0402, -10.746) (23.8086, -11.0085) (23.6151, -11.0085) knots 0 0 0 1 2 2 2
  spline S207 degree 2 poles (23.6151, -11.0085) (23.4165, -11.0085) (23.189, -10.7378) (23.189, -10.5052) knots 0 0 0 1 2 2 2
  spline S208 degree 2 poles (23.189, -10.5052) (23.189, -10.2664) (23.4237, -10.0019) (23.6151, -10.0019) knots 0 0 0 1 2 2 2
  spline S209 degree 2 poles (23.6151, -10.0019) (23.8086, -10.0019) (24.0402, -10.2654) (24.0402, -10.5052) knots 0 0 0 1 2 2 2
  spline S210 degree 2 poles (23.8745, -10.5052) (23.8745, -10.3199) (23.7396, -10.1398) (23.6151, -10.1398) knots 0 0 0 1 2 2 2
  spline S211 degree 2 poles (23.6151, -10.1398) (23.4906, -10.1398) (23.3547, -10.3199) (23.3547, -10.5052) knots 0 0 0 1 2 2 2
  spline S212 degree 2 poles (23.3547, -10.5052) (23.3547, -10.6853) (23.4906, -10.8705) (23.6151, -10.8705) knots 0 0 0 1 2 2 2
  spline S213 degree 2 poles (23.6151, -10.8705) (23.7386, -10.8705) (23.8745, -10.6884) (23.8745, -10.5052) knots 0 0 0 1 2 2 2
  line L143 (24.3685, -10.9817) -> (24.2079, -10.9817)
  line L144 (24.2079, -10.9817) -> (24.2079, -9.6551)
  line L145 (24.2079, -9.6551) -> (24.3685, -9.6551)
  line L146 (24.3685, -9.6551) -> (24.3685, -10.9817)
  point P0 (76.2, -5.7603)
  constraints: 2 other
extrude "Extrusion6" cut sketch "Sketch7" against normal blind 0.2286
extrude "Extrusion7" cut sketch "Sketch8" against normal blind 0.2286
body "Solid1"
